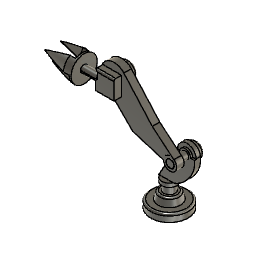
ROBO ARM_ (Autodesk Fusion 360 design; units mm, degrees)
Autodesk Fusion 360 part; units mm, degrees
sketch "Sketch1" plane through (0, 0, 0) normal (0, 0, 1) x (1, 0, 0)
  circle A0 centre (0, 0) radius 50
  dimension "d1" = 100
  constraint coincident A0.centre origin
  measures "d1" diameter of A0
extrude "Extrude1" add sketch "Sketch1" along normal blind 20 makes body 1
sketch "Sketch2" plane through (0, 0, 20) normal (0, 0, 1) x (-1, 0, 0)
  circle A0 centre (0, 0) radius 50
  circle A1 centre (0, 0) radius 30
  dimension "d4" = 60
  constraint coincident A0.centre A1.centre
  measures "d4" diameter of A1
extrude "Extrude2" add sketch "Sketch2" along normal blind 20 draft -15 contours A1 bodies 1
sketch "Sketch3" plane through (0, 0, 40) normal (0, 0, 1) x (-1, 0, 0)
  circle A0 centre (0, 0) radius 24.641
  circle A1 centre (0, 0) radius 15
  dimension "d7" = 30
  constraint coincident A0.centre A1.centre
  measures "d7" diameter of A1
extrude "Extrude3" add sketch "Sketch3" along normal blind 30 contours A1 bodies 1
sketch "Sketch4" plane through (0, 0, 70) normal (0, 0, 1) x (-1, 0, 0)
  circle A0 centre (0, 0) radius 15
  circle A1 centre (0, 0) radius 20
  dimension "d10" = 40
  constraint coincident A0.centre A1.centre
  measures "d10" diameter of A1
extrude "Extrude4" add sketch "Sketch4" against normal blind 10 bodies 1
sketch "Sketch5" plane through (0, 0, 0) normal (0, 1, 0) x (1, 0, 0)
  circle A0 centre (50, -150) radius 25
  line L0 (49.4256, -125.0066) -> (20, -140)
  line L1 (25.0278, -151.1783) -> (-20, -70)
  spline S0 degree 5 poles (20, -70) (21.0854, -70.3879) (23.2586, -71.2219) (26.5254, -72.6471) (30.8951, -74.8986) (36.3734, -78.3095) (41.8444, -82.3237) (47.2606, -86.9337) (52.539, -92.1025) (57.5599, -97.7592) (62.1862, -103.8163) (66.2778, -110.1802) (69.7089, -116.762) (72.3865, -123.4878) (74.2702, -130.3079) (75.3533, -137.1921) (75.5883, -142.738) (75.4163, -146.9166) (75.1479, -149.7106) (74.9754, -151.1098) knots 0 0 0 0 0 0 0.066667 0.133333 0.2 0.266667 0.333333 0.4 0.466667 0.533333 0.6 0.666667 0.733333 0.8 0.866667 0.933333 1 1 1 1 1 1
  line L2 (20, -70) -> (-20, -70)
  point P0 (45.2358, -85.2991)
  point P1 (69.4399, -116.6221)
  dimension "d13" = 50
  constraint coincident A0 L0.start
  constraint coincident A0 L1.start
  constraint coincident A0 S0.end
  constraint horizontal L2
  measures "d13" diameter of A0
extrude "Extrude5" add sketch "Sketch5" along normal mid plane 16 bodies 1
sketch "Sketch6" plane through (0, -8, 0) normal (0, -1, 0) x (1, 0, 0)
  arc A0 (74.9754, 151.1098) -> (25.0278, 151.1783) centre (50, 150) ccw
  line L0 (25.0278, 151.1783) -> (-20, 70)
  line L1 (-20, 70) -> (-18.3303, 70)
  line L2 (-18.3303, 70) -> (18.3303, 70)
  line L3 (18.3303, 70) -> (20, 70)
  spline S0 degree 5 poles (20, 70) (21.0854, 70.3879) (23.2586, 71.2219) (26.5254, 72.6471) (30.8951, 74.8986) (36.3734, 78.3095) (41.8444, 82.3237) (47.2606, 86.9337) (52.539, 92.1025) (57.5599, 97.7592) (62.1862, 103.8163) (66.2778, 110.1802) (69.7089, 116.762) (72.3865, 123.4878) (74.2702, 130.3079) (75.3533, 137.1921) (75.5883, 142.738) (75.4163, 146.9166) (75.1479, 149.7106) (74.9754, 151.1098) knots 0 0 0 0 0 0 0.066667 0.133333 0.2 0.266667 0.333333 0.4 0.466667 0.533333 0.6 0.666667 0.733333 0.8 0.866667 0.933333 1 1 1 1 1 1
  line L4 (4.5064, 178.602) -> (100, 178.602)
  line L5 (100, 178.602) -> (100, 150)
  line L6 (4.5064, 150) -> (4.5064, 178.602)
  arc A1 (65, 150) -> (35, 150) centre (50, 150) ccw
  line L7 (100, 150) -> (65, 150)
  line L8 (35, 150) -> (4.5064, 150)
  dimension "d16" = 30
  constraint concentric A0 A1
  constraint horizontal L4
  constraint vertical L5
  constraint horizontal L7
  constraint vertical L6
  constraint coincident A1.end L7
  constraint collinear L7 L8
  measures "d16" diameter of A1
extrude "Extrude6" cut sketch "Sketch6" against normal blind 5 contours A0 L0 S0 A1 L7 L8 bodies 1
sketch "Sketch7" plane through (0, -8, 0) normal (0, -1, 0) x (1, 0, 0)
  line L0 (35, 150) -> (24.3742, 150)
  line L1 (24.3742, 150) -> (-20, 70)
  line L2 (-20, 70) -> (-18.3303, 70)
  line L3 (-18.3303, 70) -> (18.3303, 70)
  line L4 (18.3303, 70) -> (20, 70)
  spline S0 degree 5 poles (20, 70) (21.0854, 70.3879) (23.2586, 71.2219) (26.5254, 72.6471) (30.8951, 74.8986) (36.3734, 78.3095) (41.8444, 82.3237) (47.2606, 86.9337) (52.539, 92.1025) (57.5599, 97.7592) (62.1862, 103.8163) (66.2778, 110.1802) (69.7089, 116.762) (72.3865, 123.4878) (74.2702, 130.3079) (75.3189, 136.9736) (75.5687, 142.298) (75.4407, 146.2535) (75.2273, 148.824) (75.1026, 150) knots 0 0 0 0 0 0 0.066667 0.133333 0.2 0.266667 0.333333 0.4 0.466667 0.533333 0.6 0.666667 0.733333 0.8 0.866667 0.933333 0.989419 0.989419 0.989419 0.989419 0.989419 0.989419
  line L5 (75.1026, 150) -> (65, 150)
  arc A0 (65, 150) -> (35, 150) centre (50, 150) ccw
  circle A1 centre (50, 150) radius 10
  dimension "d19" = 20
  constraint concentric A0 A1
  measures "d19" diameter of A1
extrude "Extrude7" cut sketch "Sketch7" against normal blind 40 contours A1 bodies 1
sketch "Sketch8" plane through (0, -8, 0) normal (0, -1, 0) x (1, 0, 0)
  circle A0 centre (50, 150) radius 10
  line L0 (35, 150) -> (24.3742, 150)
  line L1 (24.3742, 150) -> (-20, 70)
  line L2 (-20, 70) -> (-18.3303, 70)
  line L3 (-18.3303, 70) -> (18.3303, 70)
  line L4 (18.3303, 70) -> (20, 70)
  spline S0 degree 5 poles (20, 70) (21.0854, 70.3879) (23.2586, 71.2219) (26.5254, 72.6471) (30.8951, 74.8986) (36.3734, 78.3095) (41.8444, 82.3237) (47.2606, 86.9337) (52.539, 92.1025) (57.5599, 97.7592) (62.1862, 103.8163) (66.2778, 110.1802) (69.7089, 116.762) (72.3865, 123.4878) (74.2702, 130.3079) (75.3189, 136.9736) (75.5687, 142.298) (75.4407, 146.2535) (75.2273, 148.824) (75.1026, 150) knots 0 0 0 0 0 0 0.066667 0.133333 0.2 0.266667 0.333333 0.4 0.466667 0.533333 0.6 0.666667 0.733333 0.8 0.866667 0.933333 0.989419 0.989419 0.989419 0.989419 0.989419 0.989419
  line L5 (75.1026, 150) -> (65, 150)
  arc A1 (65, 150) -> (35, 150) centre (50, 150) ccw
  circle A2 centre (50, 150) radius 10
  dimension "d22" = 20
  constraint concentric A0 A2
  measures "d22" diameter of A2
extrude "Extrude8" add sketch "Sketch8" along normal blind 40 separate body contours A0 A2 makes body 2
sketch "Sketch9" plane through (0, 8, 0) normal (0, 1, 0) x (-1, 0, 0)
  circle A0 centre (-50, 150) radius 10
  arc A1 (-25.0278, 151.1783) -> (-74.9754, 151.1098) centre (-50, 150) ccw
  spline S0 degree 5 poles (-74.9754, 151.1098) (-75.1479, 149.7106) (-75.4163, 146.9166) (-75.5883, 142.738) (-75.3533, 137.1921) (-74.2702, 130.3079) (-72.3865, 123.4878) (-69.7089, 116.762) (-66.2778, 110.1802) (-62.1862, 103.8163) (-57.5599, 97.7592) (-52.539, 92.1025) (-47.2606, 86.9337) (-41.8444, 82.3237) (-36.3734, 78.3095) (-30.8951, 74.8986) (-26.5254, 72.6471) (-23.2586, 71.2219) (-21.0854, 70.3879) (-20, 70) knots -1 -1 -1 -1 -1 -1 -0.933333 -0.866667 -0.8 -0.733333 -0.666667 -0.6 -0.533333 -0.466667 -0.4 -0.333333 -0.266667 -0.2 -0.133333 -0.066667 0 0 0 0 0 0
  line L0 (-20, 70) -> (-18.3303, 70)
  line L1 (-18.3303, 70) -> (18.3303, 70)
  line L2 (18.3303, 70) -> (20, 70)
  line L3 (20, 70) -> (-25.0278, 151.1783)
  circle A2 centre (-50, 150) radius 20
  dimension "d25" = 40
  constraint concentric A0 A2
  measures "d25" diameter of A2
extrude "Extrude9" add sketch "Sketch9" along normal blind 15 contours A0 | A2 bodies 1
fillet "Fillet1" radius 5 1 edges at (68.6465, 23, 142.7677) on bodies 1
sketch "Sketch10" plane through (0, -48, 0) normal (0, -1, 0) x (1, 0, 0)
  circle A0 centre (50, 150) radius 10
  circle A1 centre (50, 150) radius 17.5
  dimension "d30" = 35
  constraint concentric A0 A1
  measures "d30" diameter of A1
extrude "Extrude10" add sketch "Sketch10" against normal blind 20 bodies 2
sketch "Sketch11" plane through (0, -48, 0) normal (0, -1, 0) x (1, 0, 0)
  circle A0 centre (50, 150) radius 17.5
  circle A1 centre (50, 150) radius 11
  circle A2 centre (50, 150) radius 10
  dimension "d33" = 22
  dimension "d34" = 20
  constraint concentric A0 A1
  constraint concentric A1 A2
  measures "d33" diameter of A1
  measures "d34" diameter of A2
extrude "Extrude11" cut sketch "Sketch11" against normal blind 20 contours A1 bodies 2 makes body 3 at (67.4782, -34.6667, 149.1277)
sketch "Sketch12" plane through (0, -48, 0) normal (0, -1, 0) x (1, 0, 0)
  circle A0 centre (50, 150) radius 17.5
  circle A1 centre (50, 150) radius 11
  circle A2 centre (-100, 275) radius 35
  line L0 (-124.8315, 250.3343) -> (-50, 175)
  line L1 (-50, 175) -> (32.5004, 149.8754)
  line L2 (-73.8406, 298.2527) -> (2.2352, 212.6671)
  line L3 (2.2352, 212.6671) -> (62.3107, 162.4377)
  spline S0 degree 5 poles (32.5004, 149.8754) (32.5738, 150.4893) (32.7463, 151.6954) (33.0821, 153.4389) (33.6851, 155.6318) (34.7032, 158.145) (35.9904, 160.416) (37.5465, 162.4244) (39.362, 164.1436) (41.4111, 165.5422) (43.6585, 166.5869) (46.0654, 167.246) (48.5944, 167.4943) (51.215, 167.3196) (53.9065, 166.7254) (56.6553, 165.7217) (58.8942, 164.6012) (60.5943, 163.5867) (61.737, 162.8335) (62.3107, 162.4377) knots 0 0 0 0 0 0 0.066667 0.133333 0.2 0.266667 0.333333 0.4 0.466667 0.533333 0.6 0.666667 0.733333 0.8 0.866667 0.933333 1 1 1 1 1 1
  point P0 (37.6893, 162.4377)
  point P1 (47.7061, 167.349)
  dimension "d37" = 70
  constraint coincident A2 L0.start
  constraint tangent A2 L0
  constraint coincident A0 L1.end
  constraint coincident A2 L2.start
  constraint tangent A2 L2
  constraint coincident A0 L3.end
  constraint coincident A0 P0
  constraint coincident A0 P1
  measures "d37" diameter of A2
extrude "Extrude12" add sketch "Sketch12" against normal blind 20 contours A0 A2 L0 L1 L2 L3 S0 | A2 bodies 3
sketch "Sketch13" plane through (0, -48, 0) normal (0, -1, 0) x (1, 0, 0)
  arc A0 (32.5004, 149.8754) -> (60.0607, 164.319) centre (50, 150) ccw
  line L0 (60.0607, 164.319) -> (2.2352, 212.6671)
  line L1 (2.2352, 212.6671) -> (-73.8406, 298.2527)
  arc A1 (-73.8406, 298.2527) -> (-124.8315, 250.3343) centre (-100, 275) ccw
  line L2 (-124.8315, 250.3343) -> (-50, 175)
  line L3 (-50, 175) -> (32.5004, 149.8754)
  spline S0 degree 5 poles (37.6893, 162.4377) (38.0129, 162.7902) (38.6995, 163.4852) (39.8097, 164.4491) (41.4318, 165.5519) (43.4982, 166.5124) (45.2417, 167.0177) (46.5509, 167.2419) (47.3795, 167.3251) (47.7061, 167.349) knots 0.336413 0.336413 0.336413 0.336413 0.336413 0.336413 0.4 0.466667 0.533333 0.6 0.642894 0.642894 0.642894 0.642894 0.642894 0.642894
  arc A2 (47.7061, 167.349) -> (37.6893, 162.4377) centre (50, 150) ccw
  circle A3 centre (50, 150) radius 11
  circle A4 centre (-100, 275) radius 15
  dimension "d40" = 30
  constraint concentric A1 A4
  measures "d40" diameter of A4
extrude "Extrude13" add sketch "Sketch13" along normal blind 10 contours A4 bodies 3
sketch "Sketch14" plane through (0, -58, 0) normal (0, -1, 0) x (1, 0, 0)
  circle A0 centre (-100, 275) radius 15
  line L0 (-120, 300) -> (-70, 300)
  line L1 (-70, 300) -> (-70, 250)
  line L2 (-70, 250) -> (-120, 250)
  line L3 (-120, 250) -> (-120, 300)
  constraint horizontal L0
  constraint vertical L1
  constraint horizontal L2
  constraint vertical L3
extrude "Extrude14" add sketch "Sketch14" along normal blind 20 contours A0 | L0 L1 L2 L3 bodies 3
sketch "Sketch15" plane through (-120, 0, 0) normal (-1, 0, 0) x (0, -1, 0)
  line L0 (58, 300) -> (58, 250)
  line L1 (58, 250) -> (78, 250)
  line L2 (78, 250) -> (78, 300)
  line L3 (78, 300) -> (58, 300)
  circle A0 centre (68.1608, 275) radius 10
  dimension "d45" = 20
  measures "d45" diameter of A0
extrude "Extrude15" add sketch "Sketch15" along normal blind 40 contours L2 A0 picked at (71.1394, 275) bodies 3
sketch "Sketch16" plane through (0, -28, 0) normal (0, 1, 0) x (-1, 0, 0)
  arc A0 (-37.6893, 162.4377) -> (-47.7061, 167.349) centre (-50, 150) ccw
  spline S0 degree 5 poles (-47.7061, 167.349) (-47.3795, 167.3251) (-46.5509, 167.2419) (-45.2417, 167.0177) (-43.4982, 166.5124) (-41.4318, 165.5519) (-39.8097, 164.4491) (-38.6995, 163.4852) (-38.0129, 162.7902) (-37.6893, 162.4377) knots -0.642894 -0.642894 -0.642894 -0.642894 -0.642894 -0.642894 -0.6 -0.533333 -0.466667 -0.4 -0.336413 -0.336413 -0.336413 -0.336413 -0.336413 -0.336413
  circle A1 centre (-50, 150) radius 11
  line L0 (-32.5004, 149.8754) -> (50, 175)
  line L1 (50, 175) -> (124.8315, 250.3343)
  arc A2 (124.8315, 250.3343) -> (73.8406, 298.2527) centre (100, 275) ccw
  line L2 (73.8406, 298.2527) -> (-2.2352, 212.6671)
  line L3 (-2.2352, 212.6671) -> (-60.0607, 164.319)
  arc A3 (-60.0607, 164.319) -> (-32.5004, 149.8754) centre (-50, 150) ccw
  circle A4 centre (100, 275) radius 22.5
  dimension "d48" = 45
  constraint concentric A2 A4
  measures "d48" diameter of A4
extrude "Extrude16" add sketch "Sketch16" along normal blind 20 contours A4 bodies 3
fillet "Fillet2" radius 5 1 edges at (-79.0226, -8, 266.8637) on bodies 3
fillet "Fillet3" radius 5 1 edges at (22.9735, -8.9106, 40) on bodies 1
fillet "Fillet4" radius 5 1 edges at (-46.6164, -18.0808, 20) on bodies 1
fillet "Fillet5" radius 5 2 edges at (-120, -78, 288.3932) (-95, -78, 300) on bodies 3
sketch "Sketch17" plane through (-160, 0, 0) normal (-1, 0, 0) x (0, -1, 0)
  line L0 (78, 273.2137) -> (78, 276.7863)
  arc A0 (78, 276.7863) -> (78, 273.2137) centre (68.1608, 275) ccw
  circle A1 centre (68.1608, 275) radius 35
  dimension "d59" = 70
  constraint concentric A0 A1
  measures "d59" diameter of A1
extrude "Extrude17" add sketch "Sketch17" along normal blind 20 contours L0 A0 | A1 bodies 3
sketch "Sketch18" plane through (-180, 0, 0) normal (-1, 0, 0) x (0, -1, 0)
  circle A0 centre (68.1608, 275) radius 35
  line L0 (103.1608, 275) -> (33.1608, 275)
  line L1 (68.1608, 275) -> (85.6608, 305.3109)
  line L2 (68.1608, 275) -> (111.2912, 275) construction
  line L3 (68.1608, 275) -> (108.4692, 275) construction
  line L4 (68.1608, 275) -> (50.6608, 305.3109)
  line L5 (68.1608, 275) -> (50.6608, 244.6891)
  line L6 (68.1608, 275) -> (85.6608, 244.6891)
  circle A1 centre (68.1608, 275) radius 35
  constraint horizontal L0
  constraint horizontal L2
  constraint coincident A0.centre L1.start
  constraint horizontal L3
  constraint symmetric L0 A0.centre L1.start
  constraint concentric A0 A1
  constraint coincident A0 L1.end
  constraint coincident A0 L0.start
  constraint coincident A0 L6.end
  constraint coincident A0 L5.end
  constraint coincident A0 L0.end
  constraint coincident A0 L4.end
extrude "Extrude18" cut sketch "Sketch18" against normal blind 15 contours A0 L0 L6 A1 | A0 L1 L4 A1 | A0 L0 L5 A1 bodies 3
sketch "Sketch19" plane through (-180, 0, 0) normal (-1, 0, 0) x (0, -1, 0)
  line L0 (68.1608, 275) -> (50.6608, 305.3109)
  arc A0 (50.6608, 305.3109) -> (33.1608, 275) centre (68.1608, 275) ccw
  line L1 (33.1608, 275) -> (68.1608, 275)
  circle A1 centre (68.1608, 275) radius 12.5
  dimension "d67" = 25
  constraint concentric A0 A1
  measures "d67" diameter of A1
extrude "Extrude19" cut sketch "Sketch19" against normal blind 15 contours L0 L1 A1 | L0 L1 A1 bodies 3
sketch "Sketch20" plane through (0, 0, 275) normal (0, 0, -1) x (1, 0, 0)
  line L0 (-165, 55.6608) -> (-180, 55.6608)
  line L1 (-180, 55.6608) -> (-180, 33.1608)
  line L2 (-180, 33.1608) -> (-165, 33.1608)
  line L3 (-165, 33.1608) -> (-165, 55.6608)
extrude "Extrude20" add 1 faces at (-180, -89.7952, 291.8546) along direction (-1, 0, 0) blind 80 draft -10 on bodies 3 bodies 3
extrude "Extrude21" add 1 faces at (-180, -46.5265, 291.8546) along direction (-1, 0, 0) blind 80 draft -10 on bodies 3 bodies 3
extrude "Extrude22" add 1 faces at (-180, -80.3398, 250.4277) along direction (-1, 0, 0) blind 80 draft -10 on bodies 3 bodies 3
